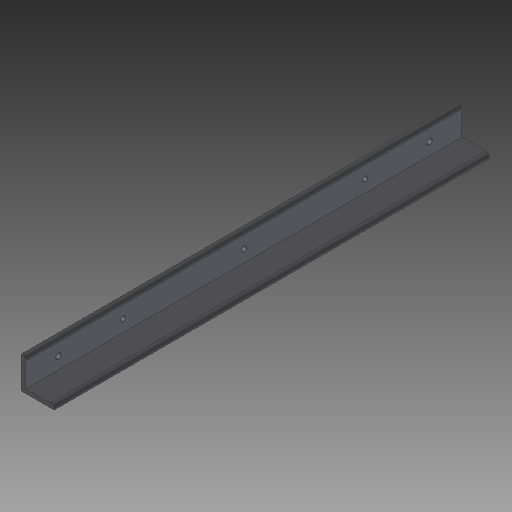
# Autodesk Inventor part: 1213_Angle Stock Bracket_V1
Saved by Autodesk Inventor 2020 (Build 240168000, 168)
## iProperties
Created: 2019-10-12
Part Number: 1213_Angle Stock Bracket_V1
Material: Aluminum
Document SubType Name: Modeling
Designer: RFLab
Density: 2.7 g/cm^3
Appearance: Satin
Mass: 135.307 g
Surface Area: 342.632 cm^2
Volume: 50.1136 cm^3
Author: RFLab
Autodesk Inventor part; units mm, degrees
ref_plane "YZ Plane" through (0, 0, 0) normal (1, 0, 0) x (0, 1, 0)
ref_plane "XZ Plane" through (0, 0, 0) normal (0, 1, 0) x (-1, 0, 0)
ref_plane "XY Plane" through (0, 0, 0) normal (0, 0, 1) x (1, 0, 0)
sketch "Sketch1" plane through (0, 0, 0) normal (0, 0, 1) x (1, 0, 0)
  line L0 (-12.7, -12.7) -> (12.7, -12.7)
  line L1 (12.7, -12.7) -> (12.7, 12.7)
  line L2 (12.7, 12.7) -> (-12.7, 12.7)
  line L3 (-12.7, 12.7) -> (-12.7, -12.7)
  line L4 (-9.525, 9.525) -> (9.525, 9.525)
  line L5 (9.525, 9.525) -> (9.525, -9.525)
  line L6 (9.525, -9.525) -> (-9.525, -9.525)
  line L7 (-9.525, -9.525) -> (-9.525, 9.525)
  arc A0 (-9.525, 9.525) -> (-12.7, 12.7) centre (-12.7, 9.525) ccw
  arc A1 (12.7, -12.7) -> (9.525, -9.525) centre (9.525, -12.7) ccw
  point P0 (0, 0)
  point P1 (-12.7, 0)
  point P2 (0, 12.7)
  dimension "d0" = 25.4
  dimension "d1" = 25.4
  dimension "d2" = 3.175
  constraints: 16 end point, 4 parallel, 4 point on circle, 4 tangent, 2 centre point, 2 midpoint, 2 perpendicular, 1 horizontal, 1 horizontal alignment, 1 vertical alignment, 3 other
  measures "d0" distance of L1.end L2.end
  measures "d1" distance of L0.end L1.end
  measures "d2" distance between parallel lines of L2 L4
extrude "Extrusion1" add sketch "Sketch1" along normal mid plane 342.9 contours L3 A0 L7 L6 A1 L0
sketch "Sketch2" plane through (-9.525, -9.525, 171.45) normal (1, 0, 0) x (0, 0, -1)
  line L0 (342.9, -3.175) -> (0, -3.175) projected
  line L1 (0, 22.225) -> (0, -3.175) projected
  line L2 (342.9, 22.225) -> (0, 22.225) projected
  line L3 (342.9, -3.175) -> (342.9, 22.225) projected
  line L4 (0, 9.525) -> (342.9, 9.525)
  point P0 (171.45, 9.525)
  point P1 (25.4, 9.525)
  point P2 (76.2, 9.525)
  point P3 (171.45, 9.525)
  point P4 (266.7, 9.525)
  point P5 (317.5, 9.525)
  dimension "d5" = 12.7
  dimension "d6" = 25.4
  dimension "d7" = 50.8
  dimension "d8" = 25.4
  dimension "d9" = 50.8
  constraints: 4 point on line, 2 end point, 2 midpoint, 1 coincident, 1 horizontal
  measures "d5" distance from line of L0.end L4
  measures "d6" distance from line of L1 point (25.4, 9.525)
  measures "d7" distance of point (25.4, 9.525) point (76.2, 9.525)
  measures "d8" distance from line of L3 point (317.5, 9.525)
  measures "d9" distance of point (317.5, 9.525) point (266.7, 9.525)
hole "Hole1" at (-9.525, 0, 146.05) at (-9.525, 0, 95.25) at (-9.525, 0, 0) at (-9.525, 0, -95.25) at (-9.525, 0, -146.05) direction (-1, 0, 0) diameter 4.5 depth 12.446 tip angle 118 clearance for "Flat Head Machine Screw (82)" size "#8" standard "Ansi Unified Screw Threads"
equation "\"d8\" = d6"
equation "\"d9\" = d7"
body "Solid1"
